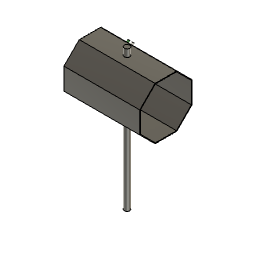
Hamme Interior Design v8 (Autodesk Fusion 360 design; units mm, degrees)
Autodesk Fusion 360 part; units mm, degrees
sketch "Sketch3" plane through (0, 0, 0) normal (0, 0, 1) x (1, 0, 0)
  line L0 (0, 0) -> (81, 0)
  line L1 (81, 0) -> (81, -58.9)
  line L2 (81, -58.9) -> (0, -58.9)
  line L3 (0, -58.9) -> (0, 0)
  line L4 (0, -58.9) -> (0, 0)
  dimension "d5" = 81
  dimension "d6" = 58.9
  dimension "d7" = 81
  constraint coincident L0.start L3.end
  constraint horizontal L0
  constraint perpendicular L0 L1
  constraint perpendicular L1 L2
  measures "d5" distance of L0.start L0.end
  measures "d6" distance of L0.end L1.end
  measures "d7" distance of L1.end L2.end
extrude "Extrude1" add sketch "Sketch3" along normal blind 1.91 makes body 1
sketch "Sketch9" plane through (0, 0, 0) normal (0, 0, 1) x (1, 0, 0)
  line L0 (63.9947, -170.6461) -> (-31.8053, -170.6461)
  line L1 (-31.8053, -170.6461) -> (-31.8053, -87.7461)
  line L2 (-31.8053, -87.7461) -> (63.9947, -87.7461)
  line L3 (63.9947, -87.7461) -> (63.9947, -170.6461)
  dimension "d17" = 95.8
  dimension "d18" = 82.9
  constraint horizontal L0
  constraint vertical L1
  constraint horizontal L2
  constraint vertical L3
  measures "d17" distance of L0.start L0.end
  measures "d18" distance of L0.start L2.end
extrude "Extrude2" add sketch "Sketch9" along normal blind 1.92 separate body makes body 2
move_body "Move1" bodies 1 to x (1, 0, 0) y (0, 1, 0) z (0, 0, 1) at (69.9573, -92.4714, 0)
move_body "Move2" bodies 2 to x (1, 0, 0) y (0, 1, 0) z (0, 0, 1) at (100.2305, 0, 1.8089)
move_body "Move3" bodies 1 2 to x (1, 0, 0) y (0, 1, 0) z (0, 0, 1) at (0, 0, 20)
move_body "Move4" bodies 1 2 to x (1, 0, 0) y (0, 1, 0) z (0, 0, 1) at (0, 2.3708, 51.5277)
sketch "Sketch12" plane through (0, 0, 0) normal (0, 0, 1) x (1, 0, 0)
  circle A0 centre (223.7981, -100.6767) radius 12.7
  dimension "d23" = 25.4
  measures "d23" diameter of A0
extrude "Extrude3" add sketch "Sketch12" along normal blind 225 separate body makes body 3
sketch "Sketch13" plane through (0, 0, 0) normal (0, 0, 1) x (1, 0, 0)
  line L0 (-0.4905, -177.4204) -> (249.5095, -177.4204)
  line L1 (249.5095, -177.4204) -> (249.5095, -277.4204)
  line L2 (249.5095, -277.4204) -> (-0.4905, -277.4204)
  line L3 (-0.4905, -277.4204) -> (-0.4905, -177.4204)
  dimension "d26" = 250
  dimension "d27" = 100
  constraint horizontal L0
  constraint vertical L1
  constraint horizontal L2
  constraint vertical L3
  measures "d26" distance of L0.start L0.end
  measures "d27" distance of L0.start L2.end
extrude "Extrude4" add sketch "Sketch13" along normal blind 3 separate body makes body 4
move_body "Move5" bodies 4 to x (1, 0, 0) y (0, 1, 0) z (0, 0, 1) at (101.658, 128.8544, 155.4559)
move_body "Move6" bodies 1 2 to x (1, 0, 0) y (0, 1, 0) z (0, 0, 1) at (90.3293, 0, 86.7072)
move_body "Move7" bodies 1 2 to x (1, 0, 0) y (0, 1, 0) z (0, 0, 1) at (-59.1191, 30, 0)
move_body "Move8" bodies 1 2 to x (1, 0, 0) y (0, 1, 0) z (0, 0, 1) at (80, 0, 0)
copy_body "CopyPasteBodies1" bodies 4 makes body 5
move_body "Move9" bodies 5 to x (1, 0, 0) y (0, 1, 0) z (0, 0, 1) at (0, -100, 0)
move_body "Move10" bodies 5 to x (1, 0, 0) y (0, 0.707107, -0.707107) z (0, 0.707107, 0.707107) at (0, -155.5592, -58.6413)
move_body "Move11" bodies 5 to x (1, 0, 0) y (0, 1, 0) z (0, 0, 1) at (0, 2.1, -0.9)
copy_body "CopyPasteBodies2" bodies 4 makes body 6
move_body "Move12" bodies 6 to x (1, 0, 0) y (0, 1, 0) z (0, 0, 1) at (0, 100, 0)
move_body "Move13" bodies 6 to x (1, 0, 0) y (0, 0.707107, 0.707107) z (0, -0.707107, 0.707107) at (0, 97.8206, 80.752)
move_body "Move14" bodies 6 to x (1, 0, 0) y (0, 1, 0) z (0, 0, 1) at (0, -2.1, -0.9)
copy_body "CopyPasteBodies3" bodies 4 makes body 7
move_body "Move15" bodies 7 to x (1, 0, 0) y (0, 1, 0) z (0, 0, 1) at (0, 70, 70)
move_body "Move16" bodies 7 to x (1, 0, 0) y (0, 0, -1) z (0, 1, 0) at (0, -207.0219, 249.89)
move_body "Move17" bodies 7 to x (1, 0, 0) y (0, 1, 0) z (0, 0, 1) at (0, 0.7, -2.3)
copy_body "CopyPasteBodies4" bodies 7 makes body 8
move_body "Move18" bodies 8 to x (1, 0, 0) y (0, 1, 0) z (0, 0, 1) at (0, -238, 0)
move_body "Move19" bodies 8 to x (1, 0, 0) y (0, 1, 0) z (0, 0, 1) at (0, -0.45, 0)
copy_body "CopyPasteBodies5" bodies 6 makes body 9
move_body "Move20" bodies 9 to x (1, 0, 0) y (0, 1, 0) z (0, 0, 1) at (0, 0, 100)
move_body "Move21" bodies 9 to x (1, 0, 0) y (0, 0, -1) z (0, 1, 0) at (0, -304.0219, 348.29)
move_body "Move22" bodies 9 to x (1, 0, 0) y (0, 1, 0) z (0, 0, 1) at (0, -2, -2)
move_body "Move23" bodies 9 to x (1, 0, 0) y (0, 1, 0) z (0, 0, 1) at (0, -0.1, -0.1)
copy_body "CopyPasteBodies6" bodies 4 makes body 10
move_body "Move24" bodies 10 to x (1, 0, 0) y (0, 1, 0) z (0, 0, 1) at (0, 0, 240)
move_body "Move25" bodies 10 to x (1, 0, 0) y (0, 1, 0) z (0, 0, 1) at (0, 0, -1.6)
copy_body "CopyPasteBodies7" bodies 9 makes body 11
move_body "Move26" bodies 11 to x (1, 0, 0) y (0, 1, 0) z (0, 0, 1) at (0, -100, 0)
move_body "Move27" bodies 11 to x (1, 0, 0) y (0, 0, -1) z (0, 1, 0) at (0, -545.4219, 244.0473)
move_body "Move28" bodies 11 to x (1, 0, 0) y (0, 1, 0) z (0, 0, 1) at (0, 2.1, 2.1)
move_body "Move29" bodies 2 to x (1, 0, 0) y (0, 1, 0) z (0, 0, 1) at (0, 0, 100)
sketch "Sketch14" plane through (0, 0, 261.9638) normal (0, 0, 1) x (-1, 0, 0)
  line L0 (-275.4354, 55.3753) -> (-179.6354, 55.3753)
  line L1 (-179.6354, 55.3753) -> (-179.6354, 138.2753)
  line L2 (-179.6354, 138.2753) -> (-275.4354, 138.2753)
  line L3 (-275.4354, 138.2753) -> (-275.4354, 55.3753)
  circle A0 centre (-240, 90) radius 10
  dimension "d59" = 20
  measures "d59" diameter of A0
extrude "Extrude5" add sketch "Sketch14" along normal blind 5 contours A0 bodies 2
move_body "Move30" bodies 2 to x (1, 0, 0) y (0, 0, 1) z (0, -1, 0) at (0, 123.6885, 400.2391)
move_body "Move31" bodies 2 to x (1, 0, 0) y (0, 1, 0) z (0, 0, 1) at (0, -85, -25)
move_body "Move32" bodies 2 to x (1, 0, 0) y (0, 1, 0) z (0, 0, 1) at (0, 5, 0)
extrude "Extrude6" add 1 faces at (233.1534, -223.2753, 287.0573) along direction (0, -1, 0) blind 5 on bodies 2 bodies 2
move_body "Move33" bodies 2 to x (1, 0, 0) y (0, 1, 0) z (0, 0, 1) at (0, 5, 0)
move_body "Move34" bodies 4 5 6 7 10 11 9 8 1 2 to x (1, 0, 0) y (0, 1, 0) z (0, 0, 1) at (0, 0, 69)
move_body "Move35" bodies 2 to x (1, 0, 0) y (0, 0, 1) z (0, -1, 0) at (-100, 258.699, 465.3956)
move_body "Move36" bodies 2 to x (1, 0, 0) y (0, 1, 0) z (0, 0, 1) at (0, 0, -25)
move_body "Move37" bodies 1 to x (1, 0, 0) y (0, 1, 0) z (0, 0, 1) at (50, 0, 0)
move_body "Move38" bodies 2 to x (1, 0, 0) y (0, 1, 0) z (0, 0, 1) at (50, 0, 0)
move_body "Move39" bodies 2 to x (1, 0, 0) y (0, 1, 0) z (0, 0, 1) at (-0.8488, -9.0219, 0)
sketch "Sketch15" plane through (0, 0, 0) normal (0, 0, 1) x (1, 0, 0)
  circle A0 centre (68.4667, 73.501) radius 5
  dimension "d65" = 10
  measures "d65" diameter of A0
extrude "Extrude7" add sketch "Sketch15" along normal blind 10 separate body makes body 12
move_body "Move40" bodies 12 to x (1, 0, 0) y (0, 1, 0) z (0, 0, 1) at (200, -175, 475)
move_body "Move41" bodies 12 to x (1, 0, 0) y (0, 1, 0) z (0, 0, 1) at (-120, -10, 0)
move_body "Move42" bodies 12 to x (1, 0, 0) y (0, 1, 0) z (0, 0, 1) at (0, 0, -10)
move_body "Move43" bodies 12 to x (1, 0, 0) y (0, 0.707107, -0.707107) z (0, 0.707107, 0.707107) at (0, -274.1396, 32.6049)
copy_body "CopyPasteBodies9" bodies 12 makes body 13
move_body "Move44" bodies 13 to x (1, 0, 0) y (0, 1, 0) z (0, 0, 1) at (0, 20, -20)
move_body "Move45" bodies 1 2 4 5 11 10 12 8 6 9 7 13 to x (1, 0, 0) y (0, 1, 0) z (0, 0, 1) at (0, 0, 150)
move_body "Move46" bodies 2 to x (1, 0, 0) y (0, 0.642788, -0.766044) z (0, 0.766044, 0.642788) at (100, -405.9497, 99.5167)
move_body "Move47" bodies 1 to x (1, 0, 0) y (0, 0.707107, -0.707107) z (0, 0.707107, 0.707107) at (-125, -394.2775, 94.0211)
extrude "Extrude8" add 1 faces at (351.1675, -81.8993, 375.4559) along direction (1, 0, 0) blind 50 on bodies 4 bodies 4 7 8 9 10 11 12 13 5 6
extrude "Extrude9" add 1 faces at (101.1675, -25.3816, 399.012) along direction (-1, 0, 0) blind 50 on bodies 4 bodies 4 9 10 11 12 13 7 8
extrude "Extrude10" add 1 faces at (101.1675, -217.6029, 512.5262) along direction (-1, 0, 0) blind 50 on bodies 4 bodies 4 11
extrude "Extrude11" add 1 faces at (101.1675, -170.4564, 591.568) along direction (-1, 0, 0) blind 50 on bodies 4 bodies 4 10
extrude "Extrude12" add 1 faces at (101.1675, -81.1993, 614.1417) along direction (-1, 0, 0) blind 50 on bodies 4 bodies 4 12 13 9
extrude "Extrude13" add 1 faces at (101.1675, 20.4376, 512.1048) along direction (-1, 0, 0) blind 50 on bodies 4 bodies 4
extrude "Extrude14" add 1 faces at (351.1675, -218.316, 511.3917) along direction (1, 0, 0) blind 50 on bodies 4 bodies 4
extrude "Extrude15" add 1 faces at (220.5259, -103.9865, 225) along direction (0, 0, 1) blind 425 on bodies 3 bodies 3 12 13 4
delete_body "RemoveBody1" bodies 2
named bodies: "Arduino", "PCB", "Stem", "LED 1", "LED 2"
